Autodesk Fusion 360 part; units mm, degrees
(part 3 of 3)
sketch "Sketch3" plane through (0, 4, 0) normal (0, 1, 0) x (-1, 0, 0)
  line L0 (-33.4664, 33.5) -> (-33.5, 33.5)
  line L1 (-33.5, 33.5) -> (-33.5, -33.5)
  line L2 (-33.5, -33.5) -> (33.5, -33.5)
  line L3 (33.5, -33.5) -> (33.5, 33.5)
  line L4 (33.5, 33.5) -> (33.4664, 33.5)
  arc A0 (33.4664, 33.5) -> (-33.4664, 33.5) centre (0, 35) ccw
  line L5 (35, -35, 5) -> (35, 35, 5)
  line L6 (33.5, 33.5, 5) -> (33.5, -33.5, 5)
  line L7 (33.5, -33.5) -> (30, -33.5)
  line L8 (30, -33.5) -> (30, 4.5)
  line L9 (30, 4.5) -> (33.5, 4.5)
  line L10 (33.5, 4.5) -> (33.5, -33.5)
  line L11 (33.5, -33.5) -> (31.5, -33.5)
  line L12 (31.5, -33.5) -> (31.5, 2)
  line L13 (31.5, 2) -> (33.5, 2)
  line L14 (33.5, 2) -> (33.5, -33.5)
  line L15 (-33.5, -33.5) -> (-30, -33.5)
  line L16 (-30, -33.5) -> (-30, 4.5)
  line L17 (-30, 4.5) -> (-33.5, 4.5)
  line L18 (-33.5, 4.5) -> (-33.5, -33.5)
  line L19 (-33.5, -33.5) -> (-31.5, -33.5)
  line L20 (-31.5, -33.5) -> (-31.5, 2)
  line L21 (-31.5, 2) -> (-33.5, 2)
  line L22 (-33.5, 2) -> (-33.5, -33.5)
  line L23 (28, -33.5) -> (7, -33.5)
  line L24 (7, -33.5) -> (7, 17.5)
  line L25 (7, 17.5) -> (28, 17.5)
  line L26 (28, 17.5) -> (28, -33.5)
  line L27 (28, -33.5) -> (23.2, -33.5)
  line L28 (23.2, -33.5) -> (23.2, -31.5)
  line L29 (23.2, -31.5) -> (28, -31.5)
  line L30 (28, -31.5) -> (28, -33.5)
  line L31 (7, -33.5) -> (11.8, -33.5)
  line L32 (11.8, -33.5) -> (11.8, -31.5)
  line L33 (11.8, -31.5) -> (7, -31.5)
  line L34 (7, -31.5) -> (7, -33.5)
  line L35 (28, 17.5) -> (23.2, 17.5)
  line L36 (23.2, 17.5) -> (23.2, 15.5)
  line L37 (23.2, 15.5) -> (28, 15.5)
  line L38 (28, 15.5) -> (28, 17.5)
  line L39 (7, 17.5) -> (11.8, 17.5)
  line L40 (11.8, 17.5) -> (11.8, 15.5)
  line L41 (11.8, 15.5) -> (7, 15.5)
  line L42 (7, 15.5) -> (7, 17.5)
  circle A1 centre (23.2, 15.5) radius 0.9
  circle A2 centre (11.8, 15.5) radius 0.9
  circle A3 centre (23.2, -31.5) radius 0.9
  circle A4 centre (11.8, -31.5) radius 0.9
  line L43 (28, 17.5) -> (7, 17.5)
  line L44 (7, 17.5) -> (7, 17.8)
  line L45 (7, 17.8) -> (28, 17.8)
  line L46 (28, 17.8) -> (28, 17.5)
  line L47 (28, 17.8) -> (28.3, 17.8)
  line L48 (28.3, 17.8) -> (28.3, 12.8)
  line L49 (28.3, 12.8) -> (28, 12.8)
  line L50 (28, 12.8) -> (28, 17.8)
  line L51 (7, 17.8) -> (6.7, 17.8)
  line L52 (6.7, 17.8) -> (6.7, 12.8)
  line L53 (6.7, 12.8) -> (7, 12.8)
  line L54 (7, 12.8) -> (7, 17.8)
  line L55 (6.7, 12.8) -> (5.7, 12.8)
  line L56 (5.7, 12.8) -> (5.7, 18.8)
  line L57 (5.7, 18.8) -> (6.7, 18.8)
  line L58 (6.7, 18.8) -> (6.7, 12.8)
  line L59 (6.7, 17.8) -> (28.3, 17.8)
  line L60 (28.3, 17.8) -> (28.3, 18.8)
  line L61 (28.3, 18.8) -> (6.7, 18.8)
  line L62 (6.7, 18.8) -> (6.7, 17.8)
  line L63 (28.3, 12.8) -> (29.3, 12.8)
  line L64 (29.3, 12.8) -> (29.3, 18.8)
  line L65 (29.3, 18.8) -> (28.3, 18.8)
  line L66 (28.3, 18.8) -> (28.3, 12.8)
  line L67 (-33.5, -33.5) -> (-7.6, -33.5)
  line L68 (-7.6, -33.5) -> (-7.6, 24.2)
  line L69 (-7.6, 24.2) -> (-33.5, 24.2)
  line L70 (-33.5, 24.2) -> (-33.5, -33.5)
  line L71 (-7.6, 24.2) -> (12, 24.2)
  line L72 (12, 24.2) -> (12, 50.7)
  line L73 (12, 50.7) -> (-7.6, 50.7)
  line L74 (-7.6, 50.7) -> (-7.6, 24.2)
  line L75 (14, 22) -> (-10, 22)
  line L76 (-10, 22) -> (-10, 53)
  line L77 (-10, 53) -> (14, 53)
  line L78 (14, 53) -> (14, 22)
  line L79 (12, 24.2) -> (9.5, 24.2)
  line L80 (9.5, 24.2) -> (9.5, 28.8)
  line L81 (9.5, 28.8) -> (12, 28.8)
  line L82 (12, 28.8) -> (12, 24.2)
  line L83 (12, 50.7) -> (9.5, 50.7)
  line L84 (9.5, 50.7) -> (9.5, 46.1)
  line L85 (9.5, 46.1) -> (12, 46.1)
  line L86 (12, 46.1) -> (12, 50.7)
  circle A5 centre (9.5, 28.8) radius 1.4
  circle A6 centre (9.5, 46.1) radius 1.4
  line L87 (7, -33.5) -> (14, -33.5)
  line L88 (14, -33.5) -> (14, -21.7)
  line L89 (14, -21.7) -> (7, -21.7)
  line L90 (7, -21.7) -> (7, -33.5)
  circle A7 centre (14, -21.7) radius 0.75
  point P0 (0, 35)
  dimension "d32" = 1.5
  dimension "d40" = 3.5
  dimension "d41" = 38
  dimension "d42" = 2
  dimension "d43" = 35.5
  dimension "d46" = 3.5
  dimension "d47" = 38
  dimension "d48" = 2
  dimension "d49" = 35.5
  dimension "d77" = 21
  dimension "d78" = 51
  dimension "d79" = 5.5
  dimension "d80" = 4.8
  dimension "d81" = 2
  dimension "d82" = 4.8
  dimension "d83" = 2
  dimension "d84" = 4.8
  dimension "d85" = 2
  dimension "d86" = 4.8
  dimension "d87" = 2
  dimension "d88" = 1.8
  dimension "d89" = 1.8
  dimension "d90" = 1.8
  dimension "d91" = 1.8
  dimension "d94" = 21
  dimension "d95" = 0.3
  dimension "d96" = 0.3
  dimension "d97" = 5
  dimension "d98" = 0.3
  dimension "d99" = 5
  dimension "d100" = 1
  dimension "d101" = 6
  dimension "d102" = 21.6
  dimension "d103" = 1
  dimension "d104" = 6
  dimension "d107" = 25.9
  dimension "d108" = 57.7
  dimension "d109" = 19.6
  dimension "d110" = 26.5
  dimension "d113" = 2.5
  dimension "d114" = 4.6
  dimension "d115" = 2.5
  dimension "d116" = 4.6
  dimension "d117" = 2.8
  dimension "d118" = 2.8
  dimension "d119" = 11.8
  dimension "d120" = 1.5
  dimension "d123" = 7
  constraint horizontal L7
  constraint vertical L8
  constraint horizontal L9
  constraint vertical L10
  constraint coincident L2.end L3.start
  constraint horizontal L11
  constraint vertical L12
  constraint horizontal L13
  constraint vertical L14
  constraint horizontal L15
  constraint vertical L16
  constraint horizontal L17
  constraint vertical L18
  constraint coincident L1.end L2.start
  constraint horizontal L19
  constraint vertical L20
  constraint horizontal L21
  constraint vertical L22
  constraint coincident P0 A0.centre
  constraint horizontal L23
  constraint vertical L24
  constraint horizontal L25
  constraint vertical L26
  constraint coincident L2 L23.start
  constraint horizontal L27
  constraint vertical L28
  constraint horizontal L29
  constraint vertical L30
  constraint horizontal L31
  constraint vertical L32
  constraint horizontal L33
  constraint vertical L34
  constraint horizontal L35
  constraint vertical L36
  constraint horizontal L37
  constraint vertical L38
  constraint horizontal L39
  constraint vertical L40
  constraint horizontal L41
  constraint vertical L42
  constraint coincident L36.end L37.start
  constraint coincident L40.end L41.start
  constraint coincident L28.end L29.start
  constraint coincident L32.end L33.start
  constraint horizontal L43
  constraint vertical L44
  constraint horizontal L45
  constraint vertical L46
  constraint horizontal L47
  constraint vertical L48
  constraint horizontal L49
  constraint vertical L50
  constraint horizontal L51
  constraint vertical L52
  constraint horizontal L53
  constraint vertical L54
  constraint horizontal L55
  constraint vertical L56
  constraint horizontal L57
  constraint vertical L58
  constraint horizontal L59
  constraint vertical L60
  constraint horizontal L61
  constraint vertical L62
  constraint horizontal L63
  constraint vertical L64
  constraint horizontal L65
  constraint vertical L66
  constraint horizontal L67
  constraint vertical L68
  constraint horizontal L69
  constraint vertical L70
  constraint horizontal L71
  constraint vertical L72
  constraint horizontal L73
  constraint vertical L74
  constraint horizontal L75
  constraint vertical L76
  constraint horizontal L77
  constraint vertical L78
  constraint horizontal L79
  constraint vertical L80
  constraint horizontal L81
  constraint vertical L82
  constraint horizontal L83
  constraint vertical L84
  constraint horizontal L85
  constraint vertical L86
  constraint coincident L80.end L81.start
  constraint coincident L84.end L85.start
  constraint horizontal L87
  constraint vertical L88
  constraint horizontal L89
  constraint vertical L90
  constraint coincident L88.end L89.start
  measures "d40" distance of L2.end L7.end
  measures "d41" distance of L2.end L9.end
  measures "d42" distance of L2.end L11.end
  measures "d43" distance of L2.end L13.end
  measures "d46" distance of L1.end L15.end
  measures "d47" distance of L1.end L17.end
  measures "d48" distance of L1.end L19.end
  measures "d49" distance of L1.end L21.end
  measures "d77" distance of L23.start L23.end
  measures "d78" distance of L23.start L25.end
  measures "d79" distance of L14 L26
  measures "d80" distance of L23.start L27.end
  measures "d81" distance of L23.start L29.end
  measures "d82" distance of L23.end L31.end
  measures "d83" distance of L23.end L33.end
  measures "d84" distance of L25.end L35.end
  measures "d85" distance of L25.end L37.end
  measures "d86" distance of L24.end L39.end
  measures "d87" distance of L24.end L41.end
  measures "d88" diameter of A1
  measures "d89" diameter of A2
  measures "d90" diameter of A3
  measures "d91" diameter of A4
  measures "d94" distance of L25.end L24.end
  measures "d95" distance of L25.end L45.end
  measures "d96" distance of L45.end L47.end
  measures "d97" distance of L45.end L49.end
  measures "d98" distance of L44.end L51.end
  measures "d99" distance of L44.end L53.end
  measures "d100" distance of L52.end L55.end
  measures "d101" distance of L52.end L57.end
  measures "d102" distance of L51.end L47.end
  measures "d103" distance of L48.end L63.end
  measures "d104" distance of L48.end L60.end
  measures "d107" distance of L1.end L67.end
  measures "d108" distance of L1.end L69.end
  measures "d109" distance of L68.end L71.end
  measures "d110" distance of L68.end L73.end
  measures "d113" distance of L71.end L79.end
  measures "d114" distance of L71.end L81.end
  measures "d115" distance of L72.end L83.end
  measures "d116" distance of L72.end L85.end
  measures "d117" diameter of A5
  measures "d118" diameter of A6
  measures "d119" distance of L23.end L89.end
  measures "d120" diameter of A7
  measures "d123" distance of L88.end L89.end
extrude "Extrude13" cut sketch "Sketch3" against normal blind 5 contours L88 L89 A7 | L88 L89 A7 bodies 1
extrude "Extrude12" add sketch "Sketch3" along normal blind 5 separate body contours L68 L69 L75 L76 L77 L78 | L68 L69 L75 L76 | L80 L81 A5 | L80 L81 A5 | L84 L85 A6 | L84 L85 A6 makes body 2 at (9.2, 4, 41.9) makes body 3 at (-8.384, 5.6667, 46.9453) makes body 4 at (-10.893, 7.3333, 28.9394)
extrude "Extrude11" add sketch "Sketch3" along normal blind 5 contours L48 L60 L63 L64 L65 L66 | L45 L47 L51 L58 L59 L60 L61 L62 L66 | L52 L55 L56 L57 L58 L62 bodies 1
extrude "Extrude10" add sketch "Sketch3" along normal blind 5 contours L28 L29 A3 | L28 L29 A3 | L32 L33 A4 | L32 L33 A4 | L36 L37 A1 | L36 L37 A1 | L40 L41 A2 | L40 L41 A2 bodies 1
extrude "Extrude5" add sketch "Sketch3" along normal blind 4 contours L1 L2 L15 L16 L17 L18 L20 L21 L67 L70 | L2 L3 L7 L8 L9 L10 L12 L13 bodies 1
sketch "Sketch4" plane through (0, 0, -35) normal (0, 0, -1) x (-1, 0, 0)
  line L0 (-35, 0) -> (35, 0)
  line L1 (35, 0) -> (35, 9)
  line L2 (35, 9) -> (-35, 9)
  line L3 (-35, 9) -> (-35, 0)
  line L4 (35, 0) -> (22, 0)
  line L5 (22, 0) -> (22, 4)
  line L6 (22, 4) -> (35, 4)
  line L7 (35, 4) -> (35, 0)
  line L8 (22, 4) -> (13, 4)
  line L9 (13, 4) -> (13, 9)
  line L10 (13, 9) -> (22, 9)
  line L11 (22, 9) -> (22, 4)
  dimension "d34" = 13
  dimension "d35" = 4
  dimension "d36" = 9
  dimension "d37" = 5
  constraint horizontal L4
  constraint vertical L5
  constraint horizontal L6
  constraint vertical L7
  constraint coincident L0.end L1.start
  constraint horizontal L8
  constraint vertical L9
  constraint horizontal L10
  constraint vertical L11
  measures "d34" distance of L0.end L4.end
  measures "d35" distance of L0.end L6.end
  measures "d36" distance of L5.end L8.end
  measures "d37" distance of L5.end L10.end
extrude "Extrude4" cut sketch "Sketch4" against normal blind 2 contours L2 L8 L9 L10 L11 bodies 1
sketch "Sketch5" plane through (0, 4, 0) normal (0, 1, 0) x (-1, 0, 0)
  line L0 (22, -33.5) -> (30, -33.5)
  line L1 (30, -33.5) -> (30, 4.5)
  line L2 (30, 4.5) -> (33.5, 4.5)
  line L3 (33.5, 4.5) -> (33.5, 33.5)
  line L4 (33.5, 33.5) -> (33.4664, 33.5)
  arc A0 (33.4664, 33.5) -> (-33.4664, 33.5) centre (0, 35) ccw
  line L5 (-33.4664, 33.5) -> (-33.5, 33.5)
  line L6 (-33.5, 33.5) -> (-33.5, 4.5)
  line L7 (-33.5, 4.5) -> (-30, 4.5)
  line L8 (-30, 4.5) -> (-30, -33.5)
  line L9 (-30, -33.5) -> (13, -33.5)
  line L10 (13, -33.5) -> (13, -35)
  line L11 (13, -35) -> (22, -35)
  line L12 (22, -35) -> (22, -33.5)
  line L13 (0, 0) -> (-1, 0)
  line L14 (-1, 0) -> (-1, 8)
  line L15 (-1, 8) -> (0, 8)
  line L16 (0, 8) -> (0, 0)
  circle A1 centre (0, 8) radius 2.05
  circle A2 centre (23.2, 15.5) radius 0.9
  circle A3 centre (23.2, -31.5) radius 0.9
  circle A4 centre (11.8, 15.5) radius 0.9
  circle A5 centre (11.8, -31.5) radius 0.9
  line L17 (6.7, 17.8) -> (6.7, 12.8)
  line L18 (6.7, 12.8) -> (5.7, 12.8)
  line L19 (5.7, 12.8) -> (5.7, 18.8)
  line L20 (5.7, 18.8) -> (29.3, 18.8)
  line L21 (29.3, 18.8) -> (29.3, 12.8)
  line L22 (29.3, 12.8) -> (28.3, 12.8)
  line L23 (28.3, 12.8) -> (28.3, 17.8)
  line L24 (28.3, 17.8) -> (6.7, 17.8)
  circle A6 centre (14, -21.7) radius 0.75
  dimension "d70" = 8
  dimension "d71" = 4.1
  constraint horizontal L13
  constraint vertical L14
  constraint horizontal L15
  constraint vertical L16
  constraint coincident L13.start L16.end
  constraint coincident L15.end L16.start
  measures "d70" distance of L13.start L15.end
  measures "d71" diameter of A1
extrude "Extrude8" cut sketch "Sketch5" against normal blind 5 contours L14 L15 L16 A1 | L14 L15 L16 A1 bodies 1
sketch "Sketch6" plane through (0, 0, 0) normal (0, -1, 0) x (1, 0, 0)
  circle A0 centre (0, 8) radius 2.05
  line L0 (-35, 35) -> (-35, -35)
  line L1 (-35, -35) -> (35, -35)
  line L2 (35, -35) -> (35, 35)
  arc A1 (35, 35) -> (-35, 35) centre (0, 35) ccw
  circle A2 centre (0, 8) radius 4
  circle A3 centre (-14, -21.7) radius 0.75
  dimension "d74" = 8
  constraint concentric A0 A2
  measures "d74" diameter of A2
extrude "Extrude9" cut sketch "Sketch6" against normal blind 3 contours A2 bodies 1
